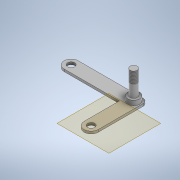
# Autodesk Inventor part: linkToActuator2
Saved by Autodesk Inventor 2021 (Build 250183000, 183)
## iProperties
Created: 2020-12-19
Part Number: linkToActuator2
Material: Generic
Document SubType Name: Modeling
Designer: awitc
Density: 1 g/cm^3
Appearance: Smooth - Medium Gray
Author: awitc
Autodesk Inventor part; units mm, degrees
ref_plane "YZ Plane" through (0, 0, 0) normal (1, 0, 0) x (0, 1, 0)
ref_plane "XZ Plane" through (0, 0, 0) normal (0, 1, 0) x (-1, 0, 0)
ref_plane "XY Plane" through (0, 0, 0) normal (0, 0, 1) x (1, 0, 0)
sketch "Sketch1" plane through (0, 0, 0) normal (0, 1, 0) x (-1, 0, 0)
  circle A0 centre (3, -13.5) radius 1.5
  circle A1 centre (29.5, -13.5) radius 1.5
  circle A2 centre (29.5, -13.5) radius 3
  circle A3 centre (3, 4.5) radius 1.5
  circle A4 centre (3, 4.5) radius 3
  line L0 (29.5, -16.5) -> (0, -16.5)
  line L1 (0, -16.5) -> (0, 4.5)
  line L2 (29.5, -10.5) -> (6, -10.5)
  line L3 (6, -10.5) -> (6, 4.5)
  point P0 (0, 0)
  dimension "d24" = 3
  dimension "d57" = 3
  dimension "d58" = 6
  dimension "d59" = 3
  dimension "d60" = 6
  constraints: 8 end point, 5 centre point, 4 point on circle, 3 tangent, 2 coincident, 1 horizontal, 1 perpendicular
  measures "d24" diameter of A0
  measures "d57" diameter of A1
  measures "d58" diameter of A2
  measures "d59" diameter of A3
  measures "d60" diameter of A4
ref_plane "Work Plane1" through (0, 1, 0) normal (0, 1, 0) x (1, 0, 0)
sketch "Sketch2" plane through (0, 1, 0) normal (0, 1, 0) x (1, 0, 0)
  line L0 (0, -4.5) -> (0, 14.5) projected
  circle A0 centre (-3, 13.5) radius 1.5 projected
  circle A1 centre (-3, 13.5) radius 1.5
  circle A2 centre (-3, 13.5) radius 2.5
  point P0 (0, 0)
  point P1 (-6, 10.5)
  dimension "d36" = 5
  constraints: 2 centre point, 2 coincident
  measures "d36" diameter of A2
extrude "Extrusion5" add sketch "Sketch2" along normal blind 2
extrude "Extrusion6" add sketch "Sketch2" along normal blind 12 and the other way blind 1 contours A0
thread "Thread2" size "M3x0.5" class "6g" standard "ANSI Metric M Profile" length 5
extrude "Extrusion8" add sketch "Sketch1" along normal blind 1
fillet "Fillet3" radius 2 1 edges at (0, 0.5, -16.5)
body "Solid4"
